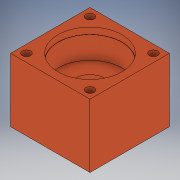
# Autodesk Inventor part: 4K heatsink bushing
Saved by Autodesk Inventor 2018 (Build 220112000, 112)
## iProperties
Created: 2019-03-19
Part Number: 4K heatsink bushing
Material: Copper
Document SubType Name: Modeling
Designer: freyja
Density: 8.94 g/cm^3
Appearance: Copper - Satin
Author: freyja
Autodesk Inventor part; units mm, degrees
ref_plane "YZ Plane" through (0, 0, 0) normal (1, 0, 0) x (0, 1, 0)
ref_plane "XZ Plane" through (0, 0, 0) normal (0, 1, 0) x (-1, 0, 0)
ref_plane "XY Plane" through (0, 0, 0) normal (0, 0, 1) x (1, 0, 0)
sketch "Sketch1" plane through (0, 0, 0) normal (0, 1, 0) x (-1, 0, 0)
  line L0 (-15.875, 15.875) -> (15.875, 15.875)
  line L1 (15.875, 15.875) -> (15.875, -15.875)
  line L2 (15.875, -15.875) -> (-15.875, -15.875)
  line L3 (-15.875, -15.875) -> (-15.875, 15.875)
  line L4 (-15.875, 15.875) -> (15.875, -15.875) construction
  line L5 (15.875, 15.875) -> (-15.875, -15.875) construction
  point P0 (0, 0)
  dimension "d0" = 31.75
  dimension "d1" = 31.75
  constraints: 12 end point, 2 midpoint, 2 parallel, 1 horizontal, 1 perpendicular
  measures "d0" distance of L1.end L2.end
  measures "d1" distance of L0.end L1.end
extrude "Extrusion1" add sketch "Sketch1" along normal mid plane 25.4
sketch "Sketch2" plane through (0, 12.7, 0) normal (0, 1, 0) x (1, 0, 0)
  point P0 (0, 0)
  point P1 (0, 0)
  constraints: 1 coincident
hole "Hole1" at (0, 12.7, 0) direction (0, -1, 0) diameter 11.5094 end through all
sketch "Sketch3" plane through (0, 12.7, 0) normal (0, 1, 0) x (1, 0, 0)
  circle A0 centre (0, 0) radius 12.7508
  dimension "d11" = 25.5016
  constraints: 1 centre point, 1 coincident
  measures "d11" diameter of A0
extrude "Extrusion2" cut sketch "Sketch3" against normal blind 11.43
sketch "Sketch4" plane through (0, 12.7, 0) normal (0, 1, 0) x (1, 0, 0)
  circle A0 centre (0, 0) radius 12.827
  dimension "d14" = 25.654
  constraints: 1 centre point, 1 coincident
  measures "d14" diameter of A0
extrude "Extrusion3" cut sketch "Sketch4" against normal blind 2.54
sketch "Sketch5" plane through (0, -12.7, 0) normal (0, -1, 0) x (1, 0, 0)
  circle A0 centre (0, 0) radius 6.3754
  dimension "d17" = 12.7508
  constraints: 1 centre point, 1 coincident
  measures "d17" diameter of A0
extrude "Extrusion4" cut sketch "Sketch5" against normal blind 11.43
sketch "Sketch6" plane through (0, -12.7, 0) normal (0, -1, 0) x (1, 0, 0)
  circle A0 centre (0, 0) radius 6.477
  dimension "d21" = 12.954
  constraints: 1 centre point, 1 coincident
  measures "d21" diameter of A0
extrude "Extrusion5" cut sketch "Sketch6" against normal blind 2.54
sketch "Sketch7" plane through (0, -12.7, 0) normal (0, -1, 0) x (1, 0, 0)
  line L0 (-12.7, 12.7) -> (12.7, 12.7) construction
  line L1 (12.7, 12.7) -> (12.7, -12.7) construction
  line L2 (12.7, -12.7) -> (-12.7, -12.7) construction
  line L3 (-12.7, -12.7) -> (-12.7, 12.7) construction
  line L4 (-12.7, 12.7) -> (12.7, -12.7) construction
  line L5 (12.7, 12.7) -> (-12.7, -12.7) construction
  point P0 (0, 0)
  dimension "d25" = 25.4
  dimension "d26" = 25.4
  constraints: 12 end point, 4 coincident, 2 midpoint, 2 parallel, 1 horizontal, 1 perpendicular
  measures "d25" distance of L1.end L2.end
  measures "d26" distance of L0.end L1.end
hole "Hole2" at (12.7, -12.7, -12.7) at (12.7, -12.7, 12.7) at (-12.7, -12.7, 12.7) at (-12.7, -12.7, -12.7) direction (0, 1, 0) diameter 3.302 end through all thread size "8-32 UNC" class "2B" standard "ANSI Unified Screw Threads"
body "Solid1"
